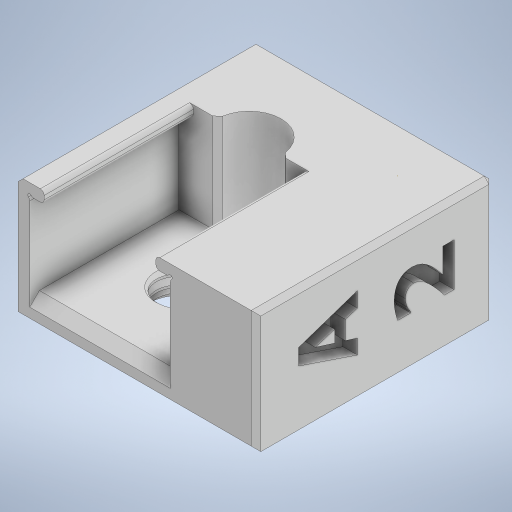
# Autodesk Inventor part: A_SampleMount_v02
Saved by Autodesk Inventor 2023 (Build 270158000, 158)
## iProperties
Created: 2021-09-08
Part Number: A_SampleMount_v02
Material: Generic
Document SubType Name: Modeling
Designer: Timo
Density: 1 g/cm^3
Appearance: Default
Author: Timo
Autodesk Inventor part; units mm, degrees
ref_plane "XZ Plane" through (0, 0, 0) normal (0, 1, 0) x (-1, 0, 0)
ref_plane "XY Plane" through (0, 0, 0) normal (0, 0, 1) x (1, 0, 0)
sketch "Sketch1" plane through (0, 0, 0) normal (0, 1, 0) x (-1, 0, 0)
  line L0 (7, -7) -> (-7, -7) construction
  line L1 (-7, -7) -> (-7, 7) construction
  line L2 (-7, 7) -> (7, 7) construction
  line L3 (7, 7) -> (7, -7) construction
  line L4 (7, -7) -> (-7, 7) construction
  line L5 (-7, -7) -> (7, 7) construction
  circle A0 centre (0, 0) radius 5 construction
  line L6 (-40.7666, 11.2) -> (45.3724, 11.2) construction
  line L7 (44.0778, -11.2) -> (-49.5298, -11.2) construction
  circle A1 centre (-11.2, -11.2) radius 5 construction
  line L8 (-16.2, 8.5) -> (8.5, 8.5)
  line L9 (8.5, 8.5) -> (8.5, -16.2)
  line L10 (8.5, -16.2) -> (-16.2, -16.2)
  line L11 (-16.2, -16.2) -> (-16.2, 8.5)
  line L12 (-7.3, 8.5) -> (7.3, 8.5) construction
  line L13 (7.3, 8.5) -> (7.3, -7) construction
  line L14 (7.3, -7) -> (-7.3, -7) construction
  line L15 (-7.3, -7) -> (-7.3, 8.5) construction
  line L16 (0, -21.68) -> (0, 16.68) construction
  circle A2 centre (0, 0) radius 2.5
  circle A3 centre (-11.2, -11.2) radius 2.5
  point P0 (0, 8.5)
  dimension "d0" = 14
  dimension "d1" = 11.2
  dimension "d2" = 11.2
  dimension "d3" = 10
  dimension "d4" = 10
  dimension "d6" = 14.6
  dimension "d7" = 1.2
  dimension "d9" = 8.5
  dimension "d10" = 8.5
  dimension "d11" = 5
  dimension "d12" = 5
  constraints: 32 end point, 6 parallel, 5 horizontal, 5 point on line, 4 centre point, 4 perpendicular, 3 coincident, 3 midpoint, 2 tangent
  measures "d0" distance of L1.end L2.end
  measures "d1" distance from line of L7 point (0, 0)
  measures "d2" distance from line of point (0, 0) L6
  measures "d3" diameter of A0
  measures "d4" diameter of A1
  measures "d6" distance between parallel lines of L15 L13
  measures "d7" distance between parallel lines of L13 L9
  measures "d9" distance from line of point (0, 0) L9
  measures "d10" distance from line of point (0, 0) L12
  measures "d11" diameter of A2
  measures "d12" diameter of A3
extrude "Extrusion1" add sketch "Sketch1" along normal blind 12
sketch "Sketch2" plane through (0, 12, 0) normal (0, 1, 0) x (1, 0, 0)
  line L0 (7.3, -8.5) -> (-7.3, -8.5)
  line L1 (-7.3, -8.5) -> (-7.3, 7)
  line L2 (-7.3, 7) -> (7.3, 7)
  line L3 (7.3, 7) -> (7.3, -8.5)
  line L4 (0, 21.14) -> (0, -13.44) projected
  line L5 (-8.5, -8.5) -> (16.2, -8.5) projected
  circle A0 centre (0, 7) radius 3.3
  point P0 (0, 0)
  point P1 (0, -8.5)
  point P2 (-3.3, 7)
  point P3 (3.3, 7)
  dimension "d15" = 7
  dimension "d16" = 14.6
  dimension "d17" = 6.6
  constraints: 8 end point, 3 point on line, 2 midpoint, 2 parallel, 1 centre point, 1 horizontal, 1 perpendicular
  measures "d15" distance from line of point (0, 0) L2
  measures "d16" distance between parallel lines of L3 L1
  measures "d17" diameter of A0
extrude "Extrusion2" cut sketch "Sketch2" against normal blind 9
chamfer "Chamfer1" distance 0.5 angle 45 2 edges at (3.3, 7.5, -7) (-3.3, 7.5, -7)
ref_plane "Work Plane1" through (11.2, 0, -11.2) normal (1, 0, 0) x (0, 1, 0)
chamfer "Chamfer2" distance 1 angle 45 2 edges at (2.5, 0, 0) (13.7, 0, -11.2)
sketch "Sketch8" plane through (11.2, 0, -11.2) normal (1, 0, 0) x (0, 1, 0)
  line L0 (0, -5) -> (0, 19.7) projected
  line L1 (0, 2.5) -> (-0.3799, 3.158)
  line L2 (-0.3799, 3.158) -> (-0.7598, 2.5)
  line L3 (-0.7598, 2.5) -> (0, 2.5)
  line L4 (-4.6678, 0) -> (14.778, 0) projected
  line L5 (-0.3464, 3.1) -> (-0.4134, 3.1)
  line L6 (-0.6299, 2.725) -> (-0.1299, 2.725) construction
  point P0 (0, 11.2)
  dimension "d51" = 2.5
  dimension "d52" = 0.5
  dimension "d53" = 30
  dimension "d54" = 60
  dimension "d55" = 3.1
  dimension "d56" = 2.725
  constraints: 10 end point, 5 point on line, 2 horizontal, 1 perpendicular
  measures "d51" distance between parallel lines of L4 L3
  measures "d52" distance of L6.start L6.end
  measures "d53" angle of L0 L1
  measures "d54" angle of L1 L2
  measures "d55" distance between parallel lines of L4 L5
  measures "d56" distance between parallel lines of L4 L6
coil "Coil1" sketch "Sketch8" operation cut axis through (11.2, 0, -11.2) along (0, 1, 0) pitch 1 turns 15 hand right contours L3 L2 L5 L1
sketch "Sketch9" plane through (0, 0, 0) normal (1, 0, 0) x (0, 1, 0)
  line L0 (3, -2.5) -> (3, 2.5) projected
  line L1 (3, 2.5) -> (3.3799, 3.158)
  line L2 (3.3799, 3.158) -> (3.7598, 2.5)
  line L3 (3.7598, 2.5) -> (3, 2.5)
  line L4 (3.1299, 2.725) -> (3.6299, 2.725) construction
  line L5 (3.3464, 3.1) -> (3.4134, 3.1)
  line L6 (3, 8.5) -> (3, -7) construction
  point P0 (0, 0)
  point P1 (3, 0)
  dimension "d65" = 2.5
  dimension "d66" = 2.725
  dimension "d67" = 3.1
  dimension "d68" = 30
  dimension "d69" = 60
  dimension "d70" = 0.5
  constraints: 10 end point, 5 point on line, 1 horizontal, 1 midpoint, 1 parallel, 1 perpendicular
  measures "d65" distance from line of point (3, 0) L3
  measures "d66" distance from line of point (3, 0) L4
  measures "d67" distance from line of point (3, 0) L5
  measures "d68" angle of L6 L1
  measures "d69" angle of L2 L1
  measures "d70" distance of L4.start L4.end
coil "Coil2" sketch "Sketch9" operation cut axis through (0, -10, 0) along (0, -1, 0) pitch 1 turns 6 hand right contours L1 L5 L2 L3
sketch "Sketch3" plane through (0, 12, 0) normal (0, 1, 0) x (1, 0, 0)
  arc A0 (8.7047, 11.046) -> (11.2, 8.7) centre (11.2, 11.2) ccw projected
  line L0 (-3.2621, 7.4986) -> (-3.8, 7) projected
  arc A1 (3.2621, 7.4986) -> (-3.2621, 7.4986) centre (0, 7) ccw projected
  line L1 (3.8, 7) -> (3.2621, 7.4986) projected
  line L2 (3.8, 7) -> (7.3, 7) projected
  line L3 (7.3, 7) -> (7.3, -8.5) projected
  line L4 (7.3, -8.5) -> (16.2, -8.5) projected
  line L5 (16.2, -8.5) -> (16.2, 16.2) projected
  line L6 (16.2, 16.2) -> (-8.5, 16.2) projected
  line L7 (-8.5, 16.2) -> (-8.5, -8.5) projected
  line L8 (-8.5, -8.5) -> (-7.3, -8.5) projected
  line L9 (-7.3, -8.5) -> (-7.3, 7) projected
  line L10 (-7.3, 7) -> (-3.8, 7) projected
  line L11 (3.8, 7) -> (7.3, 7) projected
  line L12 (5.8, 7) -> (5.8, -8.5)
  line L13 (-8.5, -8.5) -> (16.2, -8.5) projected
  line L14 (-7.3, 7) -> (-3.8, 7) projected
  line L15 (-5.8, 7) -> (-5.8, -8.5)
  line L16 (-5.8, -8.5) -> (-7.3, -8.5)
  line L17 (7.3, 7) -> (7.3, -8.5) projected
  line L18 (5.8, -8.5) -> (7.3, -8.5)
  arc A2 (13.7484, 12.9651) -> (12.8048, 13.8523) centre (11.2, 11.2) ccw projected
  point P0 (0, 0)
  dimension "d23" = 1.5
  dimension "d24" = 1.5
  constraints: 8 end point, 3 point on line, 2 vertical, 1 horizontal, 1 perpendicular, 2 other
  measures "d23" distance between parallel lines of L15 L9
  measures "d24" distance between parallel lines of L3 L12
extrude "Extrusion3" add sketch "Sketch3" along normal blind 1.2 contours L0 L10 L9 L8 L7 L6 L5 L4 L3 L2 L1 A1 | L15 L13 L9 L10 | L2 L3 L13 L12
sketch "Sketch4" plane through (-8.5, 0, 8.5) normal (0, 0, 1) x (1, 0, 0)
  line L0 (15.8, 12) -> (15.8, 3) projected
  circle A0 centre (15.8, 12) radius 0.2
  line L1 (1.2, 3) -> (1.2, 12) projected
  circle A1 centre (1.2, 12) radius 0.2
  point P0 (8.5, 0)
  dimension "d27" = 0.4
  constraints: 2 centre point, 1 equal radius
  measures "d27" diameter of A0
extrude "Extrusion4" cut sketch "Sketch4" against normal up to surface (15.5 mm away)
fillet "Fillet1" radius 0.4 4 edges at (7.1, 12, 0.75) (7.3, 11.8, 0.75) (-7.3, 11.8, 0.75) (-7.1, 12, 0.75)
fillet "Fillet2" radius 0.4 4 edges at (5.8, 13.2, 0.75) (5.8, 12, 0.75) (-5.8, 12, 0.75) (-5.8, 13.2, 0.75)
sketch "Sketch6" plane through (-8.5, 0, -16.2) normal (-1, 0, 0) x (0, 0, 1)
  line L0 (12.7, 0) -> (19.7, 0) projected
  line L1 (24.7, 0) -> (0, 0) projected
  line L2 (21.2, 0) -> (24.7, 10.2)
  line L3 (24.7, 0) -> (24.7, 13.2) projected
  line L4 (0, 13.2) -> (24.7, 13.2) projected
  point P0 (16.2, 0)
  dimension "d35" = 1.5
  dimension "d36" = 3
  constraints: 2 end point, 2 point on line
  measures "d35" distance of L2.start L0.end
  measures "d36" distance from line of L4 L2.end
extrude "Extrusion5" [suppressed]
chamfer "Chamfer3" [suppressed]
chamfer "Chamfer4" distance 0.5 angle 45 8 edges at (-8.5, 0, -3.85) (3.85, 0, -16.2) (16.2, 0, -3.85) (16.2, 6.6, 8.5) (16.2, 13.2, -3.85) (16.2, 6.6, -16.2) (3.85, 13.2, -16.2) (-8.5, 13.2, -3.85)
chamfer "Chamfer5" distance 1 angle 45 2 edges at (3.85, 0, 8.5) (0, 3, 8.5)
sketch "Sketch7" plane through (16.2, 13.2, 8.5) normal (1, 0, 0) x (0, 0, -1)
  line L0 (0, -12.2) -> (0, 0) construction
  line L1 (0, 0) -> (25, 0) construction
  line L2 (25, 0) -> (25, -12.2) construction
  line L3 (25, -12.2) -> (0, -12.2) construction
  line L4 (10.5283, -9.0215) -> (4.4283, -6.9601)
  line L5 (4.4283, -6.9601) -> (4.4283, -5.2893)
  line L6 (4.4283, -5.2893) -> (10.5283, -3.228)
  line L7 (10.5283, -3.228) -> (10.5283, -4.8049)
  line L8 (10.5283, -4.8049) -> (9.2826, -5.1855)
  line L9 (9.2826, -5.1855) -> (9.2826, -7.1035)
  line L10 (9.2826, -7.1035) -> (10.5283, -7.4891)
  line L11 (10.5283, -7.4891) -> (10.5283, -9.0215)
  line L12 (8.1753, -5.5216) -> (6.1584, -6.1445)
  line L13 (6.1584, -6.1445) -> (8.1753, -6.7723)
  line L14 (8.1753, -6.7723) -> (8.1753, -5.5216)
  line L15 (20.5717, -3.6704) -> (20.5717, -8.1539)
  line L16 (20.5717, -8.1539) -> (19.5781, -8.1539)
  spline S0 degree 2 poles (19.5781, -8.1539) (19.1234, -7.5855) (18.3226, -6.6759) (17.9617, -6.3348) knots 0 0 0 1 2 2 2
  spline S1 degree 2 poles (17.9617, -6.3348) (17.4921, -5.885) (16.7753, -5.4846) (16.3996, -5.4846) knots 0 0 0 1 2 2 2
  spline S2 degree 2 poles (16.3996, -5.4846) (15.9745, -5.4846) (15.5197, -5.9937) (15.5197, -6.4485) knots 0 0 0 1 2 2 2
  spline S3 degree 2 poles (15.5197, -6.4485) (15.5197, -6.6808) (15.6334, -7.0961) (15.7224, -7.3086) knots 0 0 0 1 2 2 2
  spline S4 degree 2 poles (15.7224, -7.3086) (15.8163, -7.5162) (16.014, -7.8128) (16.0635, -7.887) knots 0 0 0 1 2 2 2
  line L17 (16.0635, -7.887) -> (16.0635, -8.0056)
  line L18 (16.0635, -8.0056) -> (14.7337, -8.0056)
  spline S5 degree 2 poles (14.7337, -8.0056) (14.6102, -7.7486) (14.3531, -6.6512) (14.3531, -6.142) knots 0 0 0 1 2 2 2
  spline S6 degree 2 poles (14.3531, -6.142) (14.3531, -5.0545) (15.322, -3.9373) (16.1969, -3.9373) knots 0 0 0 1 2 2 2
  spline S7 degree 2 poles (16.1969, -3.9373) (16.7358, -3.9373) (17.7739, -4.4465) (18.367, -5.0347) knots 0 0 0 1 2 2 2
  spline S8 degree 2 poles (18.367, -5.0347) (18.7328, -5.4055) (19.3013, -6.1025) (19.42, -6.2557) knots 0 0 0 1 2 2 2
  line L19 (19.42, -6.2557) -> (19.42, -3.6704)
  line L20 (19.42, -3.6704) -> (20.5717, -3.6704)
  point P0 (8.5, -13.2)
  dimension "d48" = 25
  constraints: 2 coincident, 2 other
  measures "d48" distance of L0.end L1.end
extrude "Extrusion6" cut sketch "Sketch7" against normal blind 1.5
equation "\"d2\" = d1"
equation "\"d4\" = d3"
equation "\"d10\" = d9"
equation "\"d24\" = d23"
body "Solid1"
